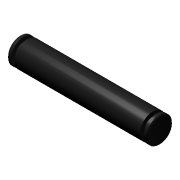
# Autodesk Inventor part: pino_a3
Saved by Autodesk Inventor 2012 SP2 (Build 160219200, 219)
## iProperties
Created: 2015-05-25
Part Number: pino_a3
Material: Aço carbono
Document SubType Name: Modeling
Designer: Projeto02
Density: 7.87 g/cm^3
Mass: 95.5272 g
Surface Area: 40.9121 cm^2
Volume: 12.1381 cm^3
Author: Projeto02
Autodesk Inventor part; units mm, degrees
ref_plane "YZ Plane" through (0, 0, 0) normal (1, 0, 0) x (0, 1, 0)
ref_plane "XZ Plane" through (0, 0, 0) normal (0, 1, 0) x (-1, 0, 0)
ref_plane "XY Plane" through (0, 0, 0) normal (0, 0, 1) x (1, 0, 0)
sketch "Esboço2" plane through (0, 0, 0) normal (1, 0, 0) x (0, 1, 0)
  circle A0 centre (0, 0) radius 7.1437
  dimension "d0" = 14.2875
  constraints: 1 centre point, 1 coincident
  measures "d0" diameter of A0
extrude "Extrusão1" add sketch "Esboço2" along normal blind 2
sketch "Esboço3" plane through (2, 0, 0) normal (1, 0, 0) x (0, 0, -1)
  circle A0 centre (0, 0) radius 7.1437 projected
  circle A1 centre (0, 0) radius 4.7625
  dimension "d3" = 9.525
  constraints: 1 centre point, 1 coincident
  measures "d3" diameter of A1
extrude "Extrusão2" add sketch "Esboço3" along normal blind 2 contours A1
sketch "Esboço4" plane through (4, 0, 0) normal (1, 0, 0) x (0, 0, -1)
  circle A0 centre (0, 0) radius 4.7625 projected
  circle A1 centre (0, 0) radius 7.1437
  dimension "d6" = 14.2875
  constraints: 1 centre point, 1 coincident
  measures "d6" diameter of A1
extrude "Extrusão3" add sketch "Esboço4" along normal blind 70 contours A0 | A1
sketch "Esboço5" plane through (74, 0, 0) normal (1, 0, 0) x (0, 0, -1)
  circle A0 centre (0, 0) radius 7.1437 projected
  circle A1 centre (0, 0) radius 4.7625
  dimension "d9" = 9.525
  constraints: 1 centre point, 1 coincident
  measures "d9" diameter of A1
extrude "Extrusão4" add sketch "Esboço5" along normal blind 2 contours A1
sketch "Esboço6" plane through (76, 0, 0) normal (1, 0, 0) x (0, 0, -1)
  circle A0 centre (0, 0) radius 4.7625 projected
  circle A1 centre (0, 0) radius 7.1437
  dimension "d12" = 14.2875
  constraints: 1 centre point, 1 coincident
  measures "d12" diameter of A1
extrude "Extrusão5" add sketch "Esboço6" along normal blind 2 contours A0 | A1
chamfer "Chanfro1" distance 0.5 angle 45 2 edges at (0, -7.1437, 0) (78, 0, 7.1437)
